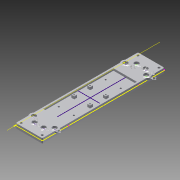
# Autodesk Inventor part: Component plate
Saved by Autodesk Inventor 2015 (Build 190159000, 159)
## iProperties
Created: 2016-01-15
Part Number: Component plate
Material: ABS Plastic
Document SubType Name: Modeling
Designer: 576994
Density: 1.06 g/cm^3
Appearance: Smooth - White
Mass: 86.1427 g
Surface Area: 328.852 cm^2
Volume: 81.2667 cm^3
Author: 576994
Autodesk Inventor part; units mm, degrees
ref_plane "YZ Plane" through (0, 0, 0) normal (1, 0, 0) x (0, 1, 0)
sketch "Sketch1" plane through (0, 0, 0) normal (0, 0, 1) x (1, 0, 0)
  line L0 (0, 0) -> (51, 0)
  line L1 (51, 0) -> (51, 235)
  line L2 (51, 235) -> (0, 235)
  line L3 (0, 235) -> (0, 0)
  dimension "d0" = 51
  dimension "d1" = 235
  constraints: 8 end point, 2 parallel, 1 horizontal, 1 perpendicular
  measures "d0" distance of L2.end L1.end
  measures "d1" distance of L1.end L0.end
extrude "Extrusion1" add sketch "Sketch1" along normal blind 5
sketch "Sketch3" plane through (0, 0, 5) normal (0, 0, 1) x (1, 0, 0)
  line L0 (0, 0) -> (51, 0) projected
  line L1 (25.5, 0) -> (25.5, 235)
  line L2 (51, 235) -> (0, 235) projected
  line L3 (0, 235) -> (0, 0) projected
  line L4 (0, 117.5) -> (51, 117.5)
  line L5 (51, 0) -> (51, 235) projected
  constraints: 4 end point, 4 midpoint
ref_plane "Work Plane1" through (25.5, 0, 5) normal (-1, 0, 0) x (0, 1, 0)
ref_plane "Work Plane2" through (0, 117.5, 5) normal (0, 1, 0) x (1, 0, 0)
sketch "Sketch4" plane through (0, 0, 5) normal (0, 0, 1) x (1, 0, 0)
  circle A0 centre (5.625, 29.5) radius 2.1
  circle A1 centre (16.875, 19.5) radius 2.1
  circle A2 centre (45.375, 29.5) radius 2.1
  circle A3 centre (34.125, 19.5) radius 2.1
  circle A4 centre (5.625, 205.5) radius 2.1
  circle A5 centre (45.375, 205.5) radius 2.1
  circle A6 centre (34.125, 215.5) radius 2.1
  circle A7 centre (16.875, 215.5) radius 2.1
  point P0 (0, 0)
  dimension "d10" = 4.2
  dimension "d11" = 4.2
  dimension "d12" = 4.2
  dimension "d13" = 4.2
  dimension "d14" = 4.2
  dimension "d15" = 4.2
  dimension "d16" = 4.2
  dimension "d17" = 4.2
  constraints: 8 centre point, 6 coincident
  measures "d10" diameter of A0
  measures "d11" diameter of A1
  measures "d12" diameter of A2
  measures "d13" diameter of A3
  measures "d14" diameter of A4
  measures "d15" diameter of A5
  measures "d16" diameter of A6
  measures "d17" diameter of A7
sketch "Sketch8" plane through (0, 0, 5) normal (0, 0, 1) x (1, 0, 0)
  line L0 (0, 0) -> (51, 0) projected
  line L1 (25.5, 0) -> (25.5, 235)
  line L2 (51, 235) -> (0, 235) projected
  line L3 (0, 235) -> (0, 0) projected
  line L4 (0, 117.5) -> (51, 117.5)
  line L5 (51, 0) -> (51, 235) projected
  line L6 (43.5, 99.5) -> (7.5, 99.5)
  line L7 (7.5, 99.5) -> (7.5, 135.5)
  line L8 (7.5, 135.5) -> (43.5, 135.5)
  line L9 (43.5, 135.5) -> (43.5, 99.5)
  line L10 (43.5, 99.5) -> (7.5, 135.5) construction
  line L11 (7.5, 99.5) -> (43.5, 135.5) construction
  line L12 (40.75, 102.25) -> (10.25, 102.25)
  line L13 (10.25, 102.25) -> (10.25, 132.75)
  line L14 (10.25, 132.75) -> (40.75, 132.75)
  line L15 (40.75, 132.75) -> (40.75, 102.25)
  line L16 (40.75, 102.25) -> (10.25, 132.75) construction
  line L17 (10.25, 102.25) -> (40.75, 132.75) construction
  line L18 (13, 105) -> (7.5, 105)
  line L19 (7.5, 105) -> (7.5, 99.5)
  line L20 (7.5, 99.5) -> (13, 99.5)
  line L21 (13, 99.5) -> (13, 105)
  line L22 (13, 105) -> (7.5, 99.5) construction
  line L23 (7.5, 105) -> (13, 99.5) construction
  line L24 (13, 130) -> (7.5, 130)
  line L25 (7.5, 130) -> (7.5, 135.5)
  line L26 (7.5, 135.5) -> (13, 135.5)
  line L27 (13, 135.5) -> (13, 130)
  line L28 (13, 130) -> (7.5, 135.5) construction
  line L29 (7.5, 130) -> (13, 135.5) construction
  line L30 (38, 105) -> (43.5, 105)
  line L31 (43.5, 105) -> (43.5, 99.5)
  line L32 (43.5, 99.5) -> (38, 99.5)
  line L33 (38, 99.5) -> (38, 105)
  line L34 (38, 105) -> (43.5, 99.5) construction
  line L35 (43.5, 105) -> (38, 99.5) construction
  line L36 (38, 130) -> (43.5, 130)
  line L37 (43.5, 130) -> (43.5, 135.5)
  line L38 (43.5, 135.5) -> (38, 135.5)
  line L39 (38, 135.5) -> (38, 130)
  line L40 (38, 130) -> (43.5, 135.5) construction
  line L41 (43.5, 130) -> (38, 135.5) construction
  point P0 (25.5, 117.5)
  dimension "d36" = 36
  dimension "d37" = 36
  dimension "d38" = 30.5
  dimension "d39" = 30.5
  constraints: 76 end point, 17 midpoint, 12 parallel, 6 horizontal, 6 perpendicular
  measures "d36" distance of L7.end L8.end
  measures "d37" distance of L6.end L7.end
  measures "d38" distance of L13.end L14.end
  measures "d39" distance of L12.end L13.end
extrude "Extrusion8" add sketch "Sketch8" along normal blind 5 contours L33 L12 L15 L30 L9 L6 | L6 L7 L18 L13 L12 L21 | L7 L8 L27 L14 L13 L24 | L33 L30 L15 L12 | L12 L13 L18 L21 | L13 L14 L27 L24 | L36 L15 L14 L39 L8 L9 | L36 L39 L14 L15
sketch "Sketch9" plane through (0, 0, 10) normal (0, 0, 1) x (1, 0, 0)
  line L0 (7.5, 99.5) -> (13, 99.5) projected
  line L1 (10.25, 99.5) -> (10.25, 105)
  line L2 (13, 105) -> (7.5, 105) projected
  line L3 (13, 99.5) -> (13, 105) projected
  line L4 (13, 102.25) -> (7.5, 102.25)
  line L5 (7.5, 99.5) -> (7.5, 105) projected
  point P0 (0, 0)
  point P1 (10.25, 102.25)
  constraints: 5 midpoint, 4 end point
hole "Hole1" at (10.25, 102.25, 10) direction (0, 0, -1) diameter 2.616 depth 5
sketch "Sketch10" plane through (0, 0, 5) normal (0, 0, 1) x (1, 0, 0)
  line L0 (0, 0) -> (51, 0) projected
  line L1 (25.5, 0) -> (25.5, 235)
  line L2 (51, 235) -> (0, 235) projected
  line L3 (0, 235) -> (0, 0) projected
  line L4 (0, 117.5) -> (51, 117.5)
  line L5 (51, 0) -> (51, 235) projected
  point P0 (0, 185)
  point P1 (0, 50)
  point P2 (51, 50)
  point P3 (51, 185)
  constraints: 4 end point, 4 midpoint
sketch "Sketch11" plane through (0, 0, 5) normal (0, 0, 1) x (1, 0, 0)
  point P0 (0, 0)
sketch "Sketch12" plane through (0, 0, 5) normal (0, 0, 1) x (1, 0, 0)
  line L0 (51, 50) -> (0, 50) projected
  line L1 (0, 185) -> (3, 185)
  line L2 (3, 185) -> (3, 50)
  line L3 (3, 50) -> (0, 50)
  line L4 (0, 50) -> (0, 185)
  line L5 (51, 185) -> (48, 185)
  line L6 (48, 185) -> (48, 50)
  line L7 (48, 50) -> (51, 50)
  line L8 (51, 50) -> (51, 185)
  point P0 (0, 0)
  dimension "d51" = 3
  dimension "d52" = 3
  constraints: 16 end point, 4 parallel, 2 horizontal, 2 perpendicular, 2 point on line
  measures "d51" distance of L2.end L3.end
  measures "d52" distance of L7.end L6.end
extrude "Extrusion9" add sketch "Sketch12" along normal blind 4
mirror "Mirror5" about plane through (25.5, 0, 5) normal (-1, 0, 0) of "Hole1"
mirror "Mirror6" about plane through (0, 117.5, 5) normal (0, 1, 0) of "Hole1", "Mirror5"
sketch "Sketch15" plane through (0, 0, 5) normal (0, 0, 1) x (1, 0, 0)
  circle A0 centre (45.375, 29.5) radius 4.25
  circle A1 centre (34.125, 19.5) radius 4.25
  circle A2 centre (16.875, 19.5) radius 4.25
  circle A3 centre (5.625, 29.5) radius 4.25
  circle A4 centre (5.625, 205.5) radius 4.25
  circle A5 centre (16.875, 215.5) radius 4.25
  circle A6 centre (34.125, 215.5) radius 4.25
  circle A7 centre (45.375, 205.5) radius 4.25
  line L0 (51, 0) -> (51, 50) projected
  line L1 (0, 0) -> (51, 0) projected
  circle A8 centre (45.375, 29.5) radius 2.1
  circle A9 centre (34.125, 19.5) radius 2.1
  line L2 (0, 50) -> (0, 0) projected
  line L3 (0, 235) -> (0, 185) projected
  line L4 (51, 235) -> (0, 235) projected
  line L5 (51, 185) -> (51, 235) projected
  circle A10 centre (5.625, 205.5) radius 2.1
  circle A11 centre (16.875, 215.5) radius 2.1
  circle A12 centre (34.125, 215.5) radius 2.1
  circle A13 centre (45.375, 205.5) radius 2.1
  line L6 (0, 0) -> (51, 0)
  line L7 (51, 50) -> (0, 50)
  line L8 (0, 235) -> (51, 235)
  line L9 (51, 185) -> (0, 185)
  arc A14 (51, 24.5392) -> (51, 34.4608) centre (45.375, 29.5) ccw
  arc A15 (0, 34.4608) -> (0, 24.5392) centre (5.625, 29.5) ccw
  arc A16 (0, 210.4608) -> (0, 200.5392) centre (5.625, 205.5) ccw
  arc A17 (51, 200.5392) -> (51, 210.4608) centre (45.375, 205.5) ccw
  line L10 (0, 50) -> (0, 34.4608)
  line L11 (0, 24.5392) -> (0, 0)
  line L12 (51, 0) -> (51, 24.5392)
  line L13 (51, 34.4608) -> (51, 50)
  line L14 (0, 185) -> (0, 200.5392)
  line L15 (0, 210.4608) -> (0, 235)
  line L16 (51, 235) -> (51, 210.4608)
  line L17 (51, 200.5392) -> (51, 185)
  dimension "d78" = 8.5
  dimension "d79" = 8.5
  dimension "d80" = 8.5
  dimension "d81" = 8.5
  dimension "d82" = 8.5
  dimension "d83" = 8.5
  dimension "d84" = 8.5
  dimension "d85" = 8.5
  dimension "d86" = 5.625
  dimension "d87" = 29.5
  dimension "d88" = 19.5
  dimension "d89" = 16.875
  dimension "d90" = 4.2
  dimension "d91" = 4.2
  dimension "d92" = 19.5
  dimension "d93" = 16.875
  dimension "d94" = 5.625
  dimension "d95" = 29.5
  dimension "d96" = 5.625
  dimension "d97" = 29.5
  dimension "d98" = 19.5
  dimension "d99" = 16.875
  dimension "d100" = 19.5
  dimension "d101" = 16.875
  dimension "d102" = 5.625
  dimension "d103" = 29.5
  dimension "d104" = 4.2
  dimension "d105" = 4.2
  dimension "d106" = 4.2
  dimension "d107" = 4.2
  dimension "d108" = 15
  dimension "d109" = 15
  dimension "d110" = 15
  dimension "d111" = 15
  constraints: 24 end point, 18 centre point, 10 coincident, 10 parallel, 8 point on circle, 4 perpendicular, 2 horizontal
  measures "d78" diameter of A0
  measures "d79" diameter of A1
  measures "d80" diameter of A2
  measures "d81" diameter of A3
  measures "d82" diameter of A4
  measures "d83" diameter of A5
  measures "d84" diameter of A6
  measures "d85" diameter of A7
  measures "d86" distance from line of A0.centre L0
  measures "d87" distance from line of A0.centre L1
  measures "d88" distance from line of L1 A1.centre
  measures "d89" distance from line of A1.centre L0
  measures "d90" diameter of A8
  measures "d91" diameter of A9
  measures "d92" distance from line of A2.centre L1
  measures "d93" distance from line of A2.centre L2
  measures "d94" distance from line of L2 A3.centre
  measures "d95" distance from line of L1 A3.centre
  measures "d96" distance from line of A4.centre L3
  measures "d97" distance from line of A4.centre L4
  measures "d98" distance from line of L4 A5.centre
  measures "d99" distance from line of A5.centre L3
  measures "d100" distance from line of A6.centre L4
  measures "d101" distance from line of A6.centre L5
  measures "d102" distance from line of A7.centre L5
  measures "d103" distance from line of A7.centre L4
  measures "d104" diameter of A10
  measures "d105" diameter of A11
  measures "d106" diameter of A12
  measures "d107" diameter of A13
  measures "d108" diameter of A14
  measures "d109" diameter of A15
  measures "d110" diameter of A16
  measures "d111" diameter of A17
extrude "Extrusion11" add sketch "Sketch15" along normal blind 4 contours L1 L2 L7 L0 | L0 A14 | A15 L2 | L4 L5 L9 L3 | L3 A16 | A17 L5
sketch "Sketch16" plane through (5.625, 29.5, 5) normal (0, 0, 1) x (1, 0, 0)
  circle A0 centre (11.25, -10) radius 2.1
  circle A1 centre (0, 0) radius 2.1
  circle A2 centre (28.5, -10) radius 2.1
  circle A3 centre (39.75, 0) radius 2.1
  circle A4 centre (39.75, 176) radius 2.1
  circle A5 centre (28.5, 186) radius 2.1
  circle A6 centre (11.25, 186) radius 2.1
  circle A7 centre (0, 176) radius 2.1
  line L0 (-5.625, -4.9608) -> (-5.625, -29.5) projected
  line L1 (-5.625, -29.5) -> (45.375, -29.5) projected
  line L2 (45.375, -29.5) -> (45.375, -4.9608) projected
  line L3 (45.375, 4.9608) -> (45.375, 20.5) projected
  line L4 (-5.625, 205.5) -> (-5.625, 180.9608) projected
  line L5 (45.375, 205.5) -> (-5.625, 205.5) projected
  line L6 (45.375, 180.9608) -> (45.375, 205.5) projected
  dimension "d115" = 4.2
  dimension "d116" = 4.2
  dimension "d117" = 4.2
  dimension "d118" = 4.2
  dimension "d119" = 5.625
  dimension "d120" = 29.5
  dimension "d121" = 19.5
  dimension "d122" = 34.125
  dimension "d123" = 19.5
  dimension "d124" = 16.875
  dimension "d125" = 4.2
  dimension "d126" = 4.2
  dimension "d127" = 5.625
  dimension "d128" = 29.5
  dimension "d129" = 4.2
  dimension "d130" = 4.2
  dimension "d131" = 5.625
  dimension "d132" = 29.5
  dimension "d133" = 19.5
  dimension "d134" = 34.125
  dimension "d135" = 19.5
  dimension "d136" = 16.875
  dimension "d137" = 5.625
  dimension "d138" = 29.5
  constraints: 8 centre point
  measures "d115" diameter of A0
  measures "d116" diameter of A1
  measures "d117" diameter of A4
  measures "d118" diameter of A5
  measures "d119" distance from line of A1.centre L0
  measures "d120" distance from line of A1.centre L1
  measures "d121" distance from line of A0.centre L1
  measures "d122" distance from line of A0.centre L2
  measures "d123" distance from line of L1 A2.centre
  measures "d124" distance from line of A2.centre L2
  measures "d125" diameter of A2
  measures "d126" diameter of A3
  measures "d127" distance from line of L3 A3.centre
  measures "d128" distance from line of A3.centre L1
  measures "d129" diameter of A6
  measures "d130" diameter of A7
  measures "d131" distance from line of A7.centre L4
  measures "d132" distance from line of A7.centre L5
  measures "d133" distance from line of L5 A6.centre
  measures "d134" distance from line of A6.centre L6
  measures "d135" distance from line of L5 A5.centre
  measures "d136" distance from line of A5.centre L6
  measures "d137" distance from line of L6 A4.centre
  measures "d138" distance from line of L5 A4.centre
extrude "Extrusion12" cut sketch "Sketch16" against normal blind 5
ref_plane "Work Plane5" through (0, 235, 5) normal (0.7071, 0, -0.7071) x (0, -1, 0)
sketch "Sketch18" plane through (0, 235, 5) normal (0.7071, 0, -0.7071) x (0, -1, 0)
  ellipse E0 centre (29.5, -3.9775) end of major axis (37, -3.9775) minor radius 5.3033 (34.4608, 0) -> (24.5392, 0) ccw projected
  line L0 (34.4608, 0) -> (24.5392, 0)
  point P0 (235, 3.5355)
  constraints: 2 end point, 1 horizontal, 1 other
sketch "Sketch19" plane through (0, 0, 5) normal (0, 0, -1) x (-1, 0, 0)
  line L0 (0, 233) -> (0, 2) projected
  arc A0 (0, 200.5392) -> (0, 210.4608) centre (-5.625, 205.5) ccw projected
  arc A1 (0, 200.5392) -> (0, 210.4608) centre (-5.625, 205.5) ccw
  line L1 (0, 210.4608) -> (0, 200.5392)
  line L2 (0, 235) -> (0, 0) projected
  constraints: 2 end point, 2 point on circle, 1 centre point, 1 collinear, 1 concentric
revolve "Revolution1" add sketch "Sketch19" angle 90 about axis through (0, 233, 5) along (0, -1, 0)
mirror "Mirror7" about plane through (0, 117.5, 5) normal (0, 1, 0) of "Revolution1"
mirror "Mirror8" about plane through (25.5, 0, 5) normal (-1, 0, 0) of "Revolution1", "Mirror7"
sketch "Sketch20" plane through (0, 0, 5) normal (0, 0, 1) x (1, 0, 0)
  circle A0 centre (10.5, 72.5) radius 1.6 projected
  circle A1 centre (39.5, 72.5) radius 1.6 projected
  circle A2 centre (10.5, 162.5) radius 1.6 projected
  circle A3 centre (39.5, 162.5) radius 1.6 projected
  point P0 (0, 0)
extrude "Extrusion13" cut sketch "Sketch20" against normal blind 5
sketch "Sketch21" plane through (0, 0, 9) normal (0, 0, 1) x (1, 0, 0)
  circle A0 centre (5.2, 5.2) radius 2.1
  line L0 (0, 0) -> (51, 0) projected
  line L1 (0, 24.5392) -> (0, 0) projected
  line L2 (25.5, 0) -> (25.5, 235) projected
  line L3 (0, 117.5) -> (51, 117.5) projected
  circle A1 centre (45.8, 5.2) radius 2.1
  circle A2 centre (5.2, 229.8) radius 2.1
  circle A3 centre (45.8, 229.8) radius 2.1
  dimension "d150" = 4.2
  dimension "d153" = 5.2
  dimension "d154" = 5.2
  constraints: 4 centre point, 3 symmetric about line, 3 other
  measures "d150" diameter of A0
  measures "d153" distance from line of L1 A0.centre
  measures "d154" distance from line of A0.centre L0
extrude "Extrusion14" cut sketch "Sketch21" against normal blind 9
fillet "Fillet3" radius 2 4 edges at (0, 0, 4.5) (51, 0, 4.5) (0, 235, 4.5) (51, 235, 4.5)
body "Solid1"
